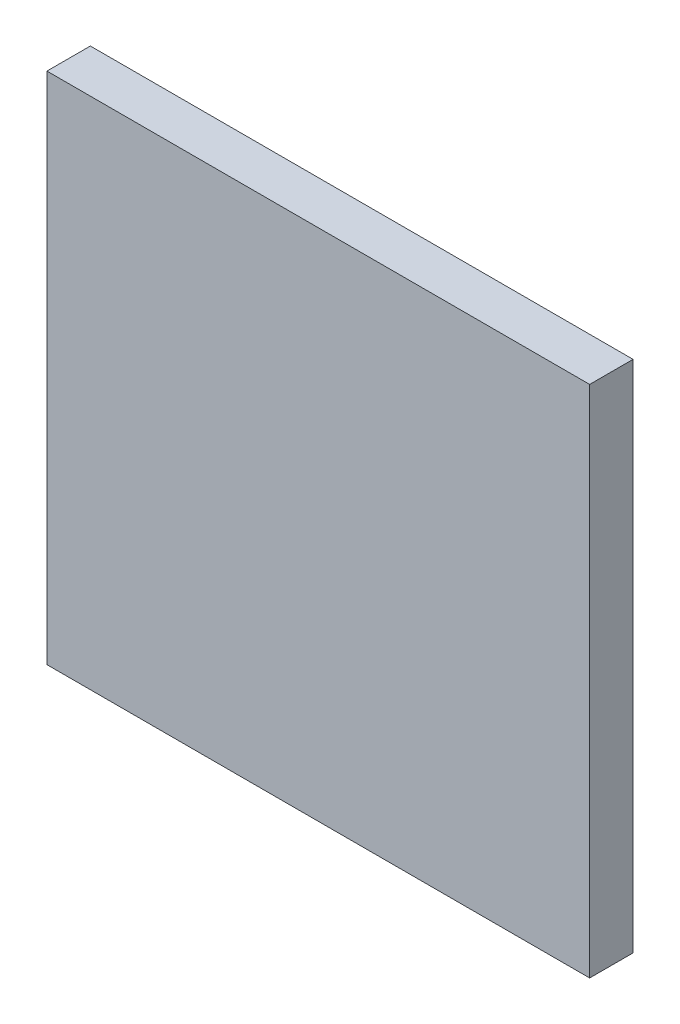
# Autodesk Inventor part: frameTop
Saved by Autodesk Inventor 2020.2 (Build 242310000, 310)
## iProperties
Created: 2020-01-07
Part Number: frameTop
Material: Generic
Document SubType Name: Modeling
Designer: steele
Density: 1 g/cm^3
Appearance: Default
Author: steele
Autodesk Inventor part; units mm, degrees
ref_plane "YZ Plane" through (0, 0, 0) normal (1, 0, 0) x (0, 1, 0)
ref_plane "XZ Plane" through (0, 0, 0) normal (0, 1, 0) x (-1, 0, 0)
ref_plane "XY Plane" through (0, 0, 0) normal (0, 0, 1) x (1, 0, 0)
ref_plane "Work Plane1" through (0, 0, 0) normal (0, 0, 1) x (1, 0, 0)
sketch "Sketch1" plane through (0, 0, 0) normal (0, 0, 1) x (1, 0, 0)
  line L0 (-53.975, -75.184) -> (-79.375, -75.184) projected
  line L1 (-53.975, -68.834) -> (-53.975, -75.184) projected
  line L2 (-79.375, -68.834) -> (-53.975, -68.834) projected
  line L3 (-79.375, -75.184) -> (-79.375, -68.834) projected
  line L4 (0, 0) -> (-79.375, 0)
  line L5 (-79.375, 0) -> (-79.375, -75.184)
  line L6 (-79.375, -75.184) -> (0, -75.184)
  line L7 (0, -75.184) -> (0, 0)
  constraints: 8 end point, 2 parallel, 1 horizontal, 1 perpendicular
extrude "Extrusion1" add sketch "Sketch1" along normal blind 6.35
body "Solid1"
